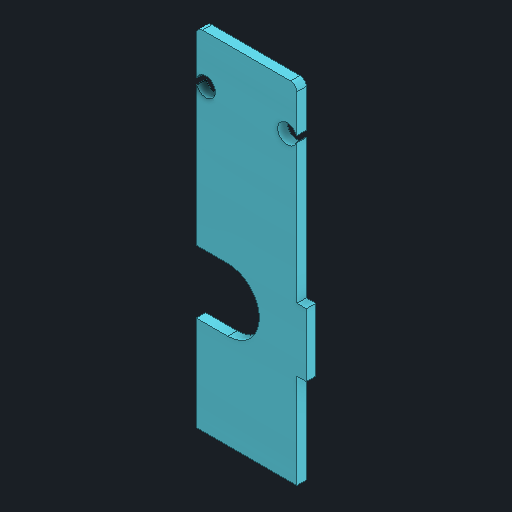
# Autodesk Inventor part: tibea_inside_steel
Saved by Autodesk Inventor 2026 (Build 300175000, 175)
## iProperties
Created: 2026-04-23
Part Number: tibea_inside_steel
Material: Сталь
Document SubType Name: Modeling
Designer: user
Density: 7.85 g/cm^3
Appearance: Серо-синий
Mass: 74.2186 g
Surface Area: 73.5434 cm^2
Volume: 9.4546 cm^3
Author: user
Autodesk Inventor part; units mm, degrees
ref_plane "YZ Plane" through (0, 0, 0) normal (1, 0, 0) x (0, 1, 0)
ref_plane "XZ Plane" through (0, 0, 0) normal (0, 1, 0) x (-1, 0, 0)
ref_plane "XY Plane" through (0, 0, 0) normal (0, 0, 1) x (1, 0, 0)
sketch "Эскиз1" plane through (0, 0, 0) normal (0, 0, 1) x (1, 0, 0)
  line L0 (0, 0) -> (-31.9, 0)
  line L1 (-29.9, 110) -> (-2, 110)
  arc A0 (-21.9, 30) -> (-21.9, 50) centre (-21.9, 40) ccw
  line L2 (-21.9, 30) -> (-31.9, 30)
  line L3 (-21.9, 50) -> (-31.9, 50)
  line L4 (0, 30) -> (3, 30)
  line L5 (3, 30) -> (3, 50)
  line L6 (3, 50) -> (0, 50)
  line L7 (-31.9, 0) -> (-31.9, 30)
  line L8 (0, 30) -> (0, 0)
  arc A1 (-31.7314, 94) -> (-31.7314, 96) centre (-28.85, 95) ccw
  line L9 (-15.95, 107.7071) -> (-15.95, 80.3284)
  line L10 (-31.9, 96) -> (-31.7314, 96)
  line L11 (-31.7314, 94) -> (-31.9, 94)
  line L12 (-32.5539, 95) -> (-24.186, 95)
  line L13 (-31.9, 50) -> (-31.9, 94)
  line L14 (-31.9, 96) -> (-31.9, 108)
  arc A2 (-0.1686, 96) -> (-0.1686, 94) centre (-3.05, 95) ccw
  line L15 (0, 96) -> (-0.1686, 96)
  line L16 (-0.1686, 94) -> (0, 94)
  line L17 (0.6539, 95) -> (-7.714, 95)
  line L18 (0, 108) -> (0, 96)
  line L19 (0, 94) -> (0, 50)
  arc A3 (-29.9, 110) -> (-31.9, 108) centre (-29.9, 108) ccw
  arc A4 (0, 108) -> (-2, 110) centre (-2, 108) ccw
  point P0 (-31.9, 110)
  point P1 (0, 110)
  dimension "d0" = 31.9
  dimension "d1" = 40
  dimension "d2" = 70
  dimension "d3" = 20
  dimension "d4" = 3
  dimension "d7" = 55
  dimension "d8" = 6.1
  dimension "d9" = 2
  dimension "d10" = 2
  constraints: 40 end point, 11 parallel, 11 tangent, 10 point on circle, 9 perpendicular, 7 point on line, 7 symmetric about line, 5 centre point, 5 horizontal, 2 collinear, 1 coincident, 1 equal radius, 1 vertical, 1 other
  measures "d0" distance of point (-31.9, 110) point (0, 110)
  measures "d1" distance from line of L0 A0.centre
  measures "d2" distance from line of L1 A0.centre
  measures "d3" diameter of A0
  measures "d4" distance of L4.start L4.end
  measures "d7" vertical distance of A0.centre A1.centre
  measures "d8" diameter of A1
  measures "d9" distance between parallel lines of L11 L10
  measures "d10" radius of A3
extrude "Выдавливание1" add sketch "Эскиз1" along normal blind 3
equation "\"d0\" = -2 * thickness_profile_tibea + hight_profile_tibea - tolerance_plazma"
equation "\"d3\" = d_main_shaft"
equation "\"d4\" = thickness_steel"
equation "\"d8\" = d_main_screw_holes"
equation "\"d5\" = thickness_steel"
equation "\"tolerance_plazma\" = 0.1"
equation "\"d_main_screw_holes\" = 6.1"
equation "\"d_main_shaft\" = 20"
equation "\"thickness_profile_tibea\" = 4"
equation "\"thickness_steel\" = 3"
equation "\"thickness_profile_femur\" = 3"
equation "\"width_shaft_shift\" = 35"
equation "\"width_flattened_surface\" = 12"
equation "\"hight_profile_tibea\" = 40"
